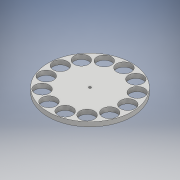
# Autodesk Inventor part: レスキューキット投下機構
Saved by Autodesk Inventor 2018 (Build 220112000, 112)
## iProperties
Created: 2018-08-16
Part Number: レスキューキット投下機構
Material: 一般
Document SubType Name: Modeling
Designer: shun2
Density: 1 g/cm^3
Appearance: 既定
Author: shun2
Autodesk Inventor part; units mm, degrees
ref_plane "YZ Plane" through (0, 0, 0) normal (1, 0, 0) x (0, 1, 0)
ref_plane "XZ Plane" through (0, 0, 0) normal (0, 1, 0) x (-1, 0, 0)
ref_plane "XY Plane" through (0, 0, 0) normal (0, 0, 1) x (1, 0, 0)
sketch "スケッチ1" plane through (0, 0, 0) normal (0, 0, 1) x (1, 0, 0)
  circle A0 centre (65, 55.362) radius 52
  circle A1 centre (65, 55.362) radius 52
  circle A2 centre (65, 97.362) radius 9
  circle A3 centre (45.4816, 92.5511) radius 9
  circle A4 centre (30.4347, 79.2207) radius 9
  circle A5 centre (23.3062, 60.4245) radius 9
  circle A6 centre (25.7293, 40.4686) radius 9
  circle A7 centre (37.1488, 23.9245) radius 9
  circle A8 centre (54.9487, 14.5824) radius 9
  circle A9 centre (75.0513, 14.5824) radius 9
  circle A10 centre (92.8512, 23.9245) radius 9
  circle A11 centre (104.2707, 40.4686) radius 9
  circle A12 centre (106.6938, 60.4245) radius 9
  circle A13 centre (99.5653, 79.2207) radius 9
  circle A14 centre (84.5184, 92.5511) radius 9
  circle A15 centre (65, 55.362) radius 1.5
  point P0 (0, 0)
  dimension "d0" = 3
  constraints: 16 centre point, 1 coincident
  measures "d0" diameter of A15
extrude "押し出し1" add sketch "スケッチ1" along normal blind 5.5
